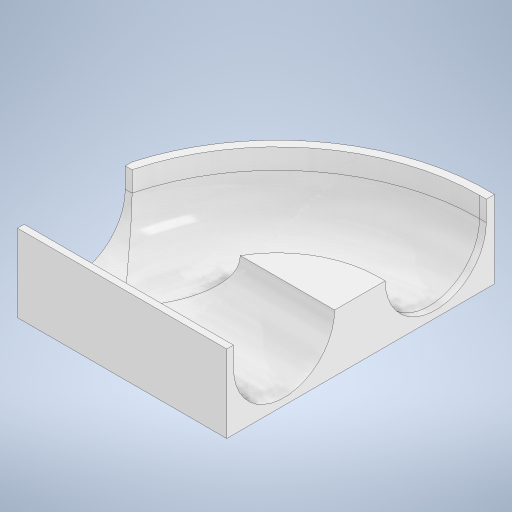
# Autodesk Inventor part: Receptor
Saved by Autodesk Inventor 2024 (Build 280153000, 153)
## iProperties
Created: 2023-05-09
Part Number: Receptor
Material: Plástico PET
Document SubType Name: Modeling
Designer: jpjoa
Density: 1.541 g/cm^3
Appearance: Branco
Author: jpjoa
Autodesk Inventor part; units mm, degrees
ref_plane "YZ Plane" through (0, 0, 0) normal (1, 0, 0) x (0, 1, 0)
ref_plane "XZ Plane" through (0, 0, 0) normal (0, 1, 0) x (-1, 0, 0)
ref_plane "XY Plane" through (0, 0, 0) normal (0, 0, 1) x (1, 0, 0)
sketch "Esboço1" plane through (0, 0, 0) normal (0, 1, 0) x (-1, 0, 0)
  line L0 (-36.0569, -1.2) -> (-1.2, -1.2)
  line L1 (-36.0569, -1.2) -> (-36.0569, -19.2)
  line L2 (-36.0569, -19.2) -> (-20.4684, -19.2)
  arc A0 (-36.0569, -28.2) -> (-20.4684, -19.2) centre (-36.0569, -10.2) ccw
  line L3 (-36.0569, -28.2) -> (-36.0569, -10.2) construction
  line L4 (-20.4684, -19.2) -> (-36.0569, -10.2) construction
  arc A1 (-36.0569, -46.2) -> (-1.2, -19.2) centre (-36.0569, -10.2) ccw
  line L5 (-36.0569, -28.2) -> (-36.0569, -46.2)
  line L6 (-1.2, -1.2) -> (-1.2, -19.2)
  line L7 (0, 0) -> (-37.2569, 0)
  line L8 (-37.2569, 0) -> (-37.2569, -20.4)
  line L9 (-37.2569, -20.4) -> (-22.7077, -20.4)
  arc A2 (-37.2569, -26.9571) -> (-22.7077, -20.4) centre (-36.0569, -10.2) ccw
  line L10 (-37.2569, -26.9571) -> (-37.2569, -47.6526)
  line L11 (0, -19.2) -> (0, 0)
  line L12 (-36.0569, -28.2) -> (-37.2569, -28.2)
  line L13 (-36.0569, -46.2) -> (-37.2569, -46.2)
  line L14 (-36.0569, -1.2) -> (-37.2569, -1.2)
  line L15 (-36.0569, -19.2) -> (-37.2569, -19.2)
  line L16 (-1.2, -19.2) -> (0, -19.2)
  line L17 (-1.2, -1.2) -> (0, -1.2)
  line L18 (-37.2569, -26.9571) -> (-37.2569, -20.4)
  line L19 (0, -20.4) -> (0, -19.2)
  arc A3 (-37.2569, -47.6526) -> (0, -20.4) centre (-36.0569, -10.2) ccw
  point P0 (-28.2626, -19.2)
  point P1 (-18.6284, 0)
  point P2 (8.0774, -19.7542)
  dimension "d19" = 60
  dimension "d21" = 18
  dimension "d22" = 1.2
  dimension "d32" = 1.2
  dimension "d33" = 1.2
  constraints: 40 end point, 8 perpendicular, 8 point on circle, 6 point on line, 5 coincident, 4 centre point, 4 vertical, 4 vertical alignment, 3 horizontal alignment, 3 midpoint, 2 collinear, 1 horizontal, 1 parallel, 3 other
  measures "d19" angle of L3 L4
  measures "d21" radial gap between concentric circles of A0 A1
  measures "d22" distance between parallel lines of L0 L7
  measures "d32" distance of L19.start L16.end
  measures "d33" distance between parallel lines of L6 L11
extrude "Extrusão2" add sketch "Esboço1" against normal blind 1.2
extrude "Extrusão3" add sketch "Esboço1" along normal blind 9 contours L14 L8 L7 L11 L17 L0 | L2 A0 L12 L10 A2 L9 L8 L15 | L9 A2 L18
extrude "Extrusão4" add sketch "Esboço1" along normal blind 12.6 contours L14 L8 L7 L11 L17 L0 | L16 L19 A3 L10 L13 A1
fillet "Arredondamento2" radius 9 7 edges at (36.6569, 0, -46.2) (14.0114, 0, -38.6605) (0.6, 0, -19.2) (18.6284, 0, -1.2) (36.6569, 0, -28.2) (27.0569, 0, -25.7885) (28.8626, 0, -19.2)
equation "\"Diâmetro_esfera\" = 18"
equation "\"Filamento\" = 0.4"
equation "\"Margem\" = 3 * Filamento"
